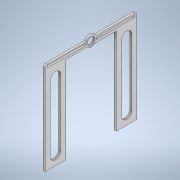
# Autodesk Inventor part: Monitor Part ReDes
Saved by Autodesk Inventor 2020.2 (Build 242310000, 310)
## iProperties
Created: 2020-05-07
Part Number: Monitor Part ReDes
Material: Generic
Document SubType Name: Modeling
Designer: Amaan Khalid
Density: 1 g/cm^3
Appearance: Default
Author: Amaan Khalid
Autodesk Inventor part; units mm, degrees
ref_plane "YZ Plane" through (0, 0, 0) normal (1, 0, 0) x (0, 1, 0)
ref_plane "XZ Plane" through (0, 0, 0) normal (0, 1, 0) x (-1, 0, 0)
ref_plane "XY Plane" through (0, 0, 0) normal (0, 0, 1) x (1, 0, 0)
sketch "Sketch1" plane through (0, 0, 0) normal (1, 0, 0) x (0, 1, 0)
  circle A0 centre (30.8347, 52.4486) radius 6.35
  line L0 (34.0644, 46.9813) -> (34.0644, -0.6437)
  line L1 (33.2311, 58.3291) -> (33.2311, 105.9541)
  line L2 (30.0561, 109.1291) -> (27.0711, 109.1291)
  arc A1 (33.2311, 105.9541) -> (30.0561, 109.1291) centre (30.0561, 105.9541) ccw
  line L3 (30.8894, -3.8187) -> (26.3644, -3.8187)
  arc A2 (30.8894, -3.8187) -> (34.0644, -0.6437) centre (30.8894, -0.6437) ccw
  line L4 (27.0711, 109.1291) -> (27.0711, 57.5631)
  line L5 (26.3644, -3.8187) -> (26.3644, 47.9388)
  line L6 (27.0711, 109.1291) -> (27.0711, 83.7291)
  line L7 (27.0711, 109.1291) -> (-79.6089, 109.1291)
  line L8 (-79.6089, 109.1291) -> (-79.6089, 83.7291)
  line L9 (-79.6089, 83.7291) -> (27.0711, 83.7291)
  line L10 (26.3644, -3.8187) -> (-80.3156, -3.8187)
  line L11 (-80.3156, -3.8187) -> (-80.3156, 21.5813)
  line L12 (26.3644, -3.8187) -> (26.3644, 21.5813)
  line L13 (26.3644, 21.5813) -> (-80.3156, 21.5813)
  circle A3 centre (30.8347, 52.4486) radius 4.7025
  point P0 (34.0644, -3.8187)
  point P1 (33.2311, 109.1291)
  dimension "d3" = 50.8
  dimension "d4" = 50.8
  dimension "d5" = 6.16
  dimension "d6" = 3.175
  dimension "d7" = 3.175
  dimension "d8" = 25.4
  dimension "d9" = 106.68
  dimension "d10" = 106.68
  dimension "d11" = 25.4
  dimension "d13" = 25.4
  dimension "d46" = 12.7
  constraints: 28 end point, 8 point on circle, 6 point on line, 4 centre point, 4 horizontal, 4 tangent, 3 perpendicular, 3 vertical, 1 coincident
  measures "d3" distance of L0.start point (34.064, -3.819)
  measures "d4" distance of L1.start point (33.231, 109.129)
  measures "d5" distance of point (33.231, 109.129) L2.end
  measures "d6" radius of A1
  measures "d7" radius of A2
  measures "d8" distance of L2.end L6.end
  measures "d9" distance of L2.end L7.end
  measures "d10" distance of L3.end L10.end
  measures "d11" distance of L10.end L11.end
  measures "d13" distance of L3.end L12.end
  measures "d46" diameter of A0
extrude "Extrusion1" add sketch "Sketch1" along normal blind 2.54 contours A0 | A0 L4 L2 A1 L1 | L0 A2 L3 L5 A0
sketch "Sketch2" plane through (2.54, 0, 0) normal (1, 0, 0) x (0, 0, -1)
  line L0 (-109.1291, 27.0711) -> (-57.5631, 27.0711) projected
  line L1 (-109.1291, 27.0711) -> (-109.1291, -79.6089)
  line L2 (-109.1291, -79.6089) -> (-83.7291, -79.6089)
  line L3 (-83.7291, -79.6089) -> (-83.7291, 27.0711)
  line L4 (-109.1291, 27.0711) -> (-83.7291, 27.0711)
  line L5 (3.8187, 26.3644) -> (3.8187, 30.8894) projected
  line L6 (3.8187, 26.3644) -> (3.8187, -80.3156)
  line L7 (3.8187, -80.3156) -> (-21.5813, -80.3156)
  line L8 (-21.5813, -80.3156) -> (-21.5813, 26.3644)
  line L9 (-47.9388, 26.3644) -> (3.8187, 26.3644) projected
  point P0 (0, 0)
  dimension "d16" = 106.68
  dimension "d17" = 25.4
  dimension "d18" = 106.68
  dimension "d19" = 25.4
  constraints: 14 end point, 3 perpendicular, 2 point on line, 2 vertical, 1 collinear, 1 horizontal
  measures "d16" distance of L0.start L1.end
  measures "d17" distance of L1.end L2.end
  measures "d18" distance of L5.start L6.end
  measures "d19" distance of L6.end L7.end
extrude "Extrusion2" add sketch "Sketch2" against normal up to surface (2.54 mm away)
sketch "Sketch3" plane through (2.54, 0, 0) normal (1, 0, 0) x (0, 0, -1)
  line L0 (-83.7291, -79.6089) -> (-83.7291, 27.0711) projected
  line L1 (-58.3291, 33.2311) -> (-105.9541, 33.2311) projected
  line L2 (-109.1291, 30.0561) -> (-109.1291, -79.6089) projected
  line L3 (-109.1291, -79.6089) -> (-83.7291, -79.6089) projected
  line L4 (-96.4291, 20.7211) -> (-96.4291, 20.7211)
  line L5 (-90.0791, 14.3711) -> (-90.0791, -66.9089)
  line L6 (-96.4291, -73.2589) -> (-96.4291, -73.2589)
  line L7 (-102.7791, -66.9089) -> (-102.7791, 14.3711)
  arc A0 (-96.4291, 20.7211) -> (-102.7791, 14.3711) centre (-96.4291, 14.3711) ccw
  arc A1 (-90.0791, 14.3711) -> (-96.4291, 20.7211) centre (-96.4291, 14.3711) ccw
  arc A2 (-102.7791, -66.9089) -> (-96.4291, -73.2589) centre (-96.4291, -66.9089) ccw
  arc A3 (-96.4291, -73.2589) -> (-90.0791, -66.9089) centre (-96.4291, -66.9089) ccw
  line L8 (-8.8813, 20.0144) -> (-8.8813, 20.0144)
  line L9 (-15.2313, 13.6644) -> (-15.2313, -67.6156)
  line L10 (-8.8813, -73.9656) -> (-8.8813, -73.9656)
  line L11 (-2.5313, -67.6156) -> (-2.5313, 13.6644)
  line L12 (-21.5813, -80.3156) -> (3.8187, -80.3156) projected
  line L13 (-47.9388, 26.3644) -> (-21.5813, 26.3644) projected
  line L14 (3.8187, -80.3156) -> (3.8187, 30.8894) projected
  line L15 (-21.5813, 26.3644) -> (-21.5813, -80.3156) projected
  arc A4 (-8.8813, 20.0144) -> (-15.2313, 13.6644) centre (-8.8813, 13.6644) ccw
  arc A5 (-2.5313, 13.6644) -> (-8.8813, 20.0144) centre (-8.8813, 13.6644) ccw
  arc A6 (-15.2313, -67.6156) -> (-8.8813, -73.9656) centre (-8.8813, -67.6156) ccw
  arc A7 (-8.8813, -73.9656) -> (-2.5313, -67.6156) centre (-8.8813, -67.6156) ccw
  circle A8 centre (-52.4486, 30.8347) radius 4.7025 projected
  line L16 (-57.1511, 30.8347) -> (-59.6911, 30.8347)
  arc A9 (-59.6911, 29.5647) -> (-59.6911, 32.1047) centre (-59.6911, 30.8347) ccw
  line L17 (-107.6225, 30.8347) -> (-105.0825, 30.8347)
  arc A10 (-105.0825, 32.1047) -> (-105.0825, 29.5647) centre (-105.0825, 30.8347) ccw
  line L18 (-105.0825, 32.1047) -> (-59.6911, 32.1047)
  line L19 (-105.0825, 29.5647) -> (-59.6911, 29.5647)
  line L20 (-47.7461, 30.8347) -> (-45.2061, 30.8347)
  arc A11 (-45.2061, 32.1047) -> (-45.2061, 29.5647) centre (-45.2061, 30.8347) ccw
  arc A12 (0.1852, 29.5647) -> (0.1852, 32.1047) centre (0.1852, 30.8347) ccw
  line L21 (0.1852, 32.1047) -> (-45.2061, 32.1047)
  line L22 (-45.2061, 29.5647) -> (0.1852, 29.5647)
  point P0 (0, 0)
  point P1 (-8.8813, 20.0144)
  point P2 (-8.8813, -73.9656)
  dimension "d26" = 6.35
  dimension "d27" = 6.35
  dimension "d28" = 6.35
  dimension "d29" = 6.35
  dimension "d30" = 6.35
  dimension "d31" = 6.35
  dimension "d32" = 6.35
  dimension "d33" = 6.35
  dimension "d34" = 6.35
  dimension "d35" = 6.35
  dimension "d36" = 2.54
  dimension "d37" = 2.54
  dimension "d38" = 2.54
  dimension "d39" = 2.54
  dimension "d40" = 2.54
  dimension "d41" = 2.54
  dimension "d43" = 2.54
  constraints: 30 end point, 26 point on circle, 21 tangent, 12 centre point, 6 equal radius, 5 horizontal, 4 parallel, 3 coincident, 2 perpendicular
  measures "d26" distance from line of L0.end L4
  measures "d27" distance between parallel lines of L0 L5
  measures "d28" distance between parallel lines of L3 L6
  measures "d29" distance between parallel lines of L2 L7
  measures "d30" radius of A0
  measures "d31" distance between parallel lines of L12 L10
  measures "d32" distance between parallel lines of L13 L8
  measures "d33" distance between parallel lines of L14 L11
  measures "d34" distance between parallel lines of L15 L9
  measures "d35" radius of A4
  measures "d36" distance of L16.start L16.end
  measures "d37" diameter of A9
  measures "d38" distance of L17.start L17.end
  measures "d39" diameter of A10
  measures "d40" distance of L20.start L20.end
  measures "d41" diameter of A11
  measures "d43" diameter of A12
extrude "Extrusion3" cut sketch "Sketch3" against normal through all contours L5 A3 A2 L7 A0 A1 | A4 A5 L11 A7 A6 L9 | L19 A10 L18 A9 | L21 A12 L22 A11
body "Solid1"
